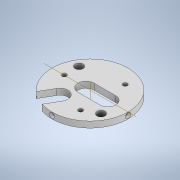
# Autodesk Inventor part: my_faceplate
Saved by Autodesk Inventor 2021 (Build 250183000, 183)
## iProperties
Created: 2020-09-14
Part Number: my_faceplate
Material: Generic
Document SubType Name: Modeling
Designer: dsouthall
Density: 1 g/cm^3
Appearance: Default
Author: dsouthall
Autodesk Inventor part; units mm, degrees
ref_plane "YZ Plane" through (0, 0, 0) normal (1, 0, 0) x (0, 1, 0)
ref_plane "XZ Plane" through (0, 0, 0) normal (0, 1, 0) x (-1, 0, 0)
ref_plane "XY Plane" through (0, 0, 0) normal (0, 0, 1) x (1, 0, 0)
sketch "Sketch1" plane through (0, 0, 0) normal (0, 1, 0) x (-1, 0, 0)
  circle A0 centre (0, 0) radius 60.325
  line L0 (0, 0) -> (60.325, 0) construction
  line L1 (0, 0) -> (-60.325, 0) construction
  line L2 (0, 0) -> (30.1625, 52.243) construction
  line L3 (0, 0) -> (-30.1625, -52.243) construction
  line L4 (0, 0) -> (-52.243, 30.1625) construction
  line L5 (0, 0) -> (17.526, 30.3559) construction
  circle A1 centre (0, 0) radius 47.625 construction
  circle A2 centre (41.2445, -23.8125) radius 6.35
  circle A3 centre (0, 0) radius 35.052 construction
  arc A4 (29.9597, 27.769) -> (9.0688, 39.8304) centre (17.526, 30.3559) ccw construction
  circle A5 centre (0, 0) radius 40.8498 construction
  circle A6 centre (40.8498, 0) radius 3.3782
  line L6 (6.5275, 36.7059) -> (18.488, 57.4221)
  line L7 (28.5245, 24.0059) -> (40.485, 44.7221)
  circle A7 centre (-20.4249, 35.3769) radius 3.3782
  circle A8 centre (-20.4249, -35.3769) radius 3.3782
  circle A9 centre (-41.2445, 23.8125) radius 6.35
  arc A10 (28.5245, 24.0059) -> (29.9597, 27.769) centre (17.526, 30.3559) ccw construction
  arc A11 (9.0688, 39.8304) -> (6.5275, 36.7059) centre (17.526, 30.3559) ccw construction
  arc A12 (6.5275, 36.7059) -> (28.5245, 24.0059) centre (17.526, 30.3559) ccw
  arc A13 (-5.8868, 3.3987) -> (6.35, -12.7) centre (6.35, 0) ccw construction
  arc A14 (-28.1432, 12.7) -> (-28.1432, -12.7) centre (-28.1432, 0) ccw
  line L8 (6.35, 12.7) -> (-28.1432, 12.7)
  line L9 (-28.1432, -12.7) -> (6.35, -12.7)
  arc A15 (6.35, 12.7) -> (-5.8868, 3.3987) centre (6.35, 0) ccw construction
  arc A16 (6.35, -12.7) -> (6.35, 12.7) centre (6.35, 0) ccw
  arc A17 (-15.4432, 0) -> (-28.1432, 12.7) centre (-28.1432, 0) ccw construction
  arc A18 (-28.1432, -12.7) -> (-15.4432, 0) centre (-28.1432, 0) ccw construction
  dimension "d0" = 120.65
  dimension "d10" = 95.25
  dimension "d1" = 60
  dimension "d2" = 120
  dimension "d3" = 30
  dimension "medium_d" = 12.7
  dimension "d12" = 70.104
  dimension "d14" = 81.6995
  dimension "small_d" = 6.7564
  dimension "d18" = 360
  dimension "d22" = 360
  dimension "large_r" = 12.7
  dimension "d25" = 0
  dimension "d26" = 6.35
  dimension "d27" = 34.4932
  dimension "d28" = 25.4
  dimension "d29" = 25.4
  constraints: 24 point on circle, 20 end point, 17 centre point, 12 tangent, 8 coincident, 6 point on line, 2 parallel, 1 collinear, 1 horizontal, 24 other
  measures "d1" angle of L2 L0
  measures "d2" angle of L3 L0
  measures "d3" angle of L4 L1
  measures "medium_d" diameter of A2
  measures "d12" diameter of A3
  measures "d14" diameter of A5
  measures "small_d" diameter of A6
  measures "large_r" radius of A12
  measures "d25" distance from line of L4 A9.centre
  measures "d26" distance of point (6.35, 0) L0.start
  measures "d27" distance of point (-28.143, 0) point (6.35, 0)
  measures "d28" diameter of A13
  measures "d29" diameter of A14
extrude "Extrusion1" add sketch "Sketch1" along normal blind 9.652 contours A0 L6 A12 L7 picked at (-0.8511, -35.9499)
ref_plane "Work Plane2" through (60.325, 0, 0) normal (-1, 0, 0) x (0, -1, 0)
ref_plane "Work Plane1" through (40.8432, 9.652, 0) normal (-1, 0, 0) x (0, -1, 0)
sketch "Sketch2" plane through (60.325, 0, 0) normal (-1, 0, 0) x (0, -1, 0)
  point P0 (0, 0)
  point P1 (-4.826, 0)
  point P2 (-9.652, 0)
  dimension "d32" = 4.826
  measures "d32" distance of point (-9.652, 0) point (-4.826, 0)
hole "Hole1" at (60.325, 4.826, 0) direction (-1, 0, 0) diameter 3.302 depth 12.2936 tip angle 118 countersink diameter 8.4328 countersink angle 82 thread size "8-32 UNC" class "2B" standard "ANSI Unified Screw Threads"
pattern_circular "Circular Pattern1" count 4 over 360 about axis through (0, 0, 0) along (0, 1, 0) of "Hole1"
equation "\"d32\" = 0.5 * thickness"
equation "\"thickness\" = 9.652"
body "Solid1"
